Joystick Holding Tab (Autodesk Fusion 360 design; units mm, degrees)
Autodesk Fusion 360 part; units mm, degrees
sketch "Sketch1" plane through (0, 0, 0) normal (0, 0, 1) x (1, 0, 0)
  line L0 (0, 0) -> (30, 0)
  line L1 (30, 0) -> (30, -10)
  line L2 (30, -10) -> (0, -10)
  line L3 (0, -10) -> (0, 0)
  line L4 (25, 0) -> (25, -10)
  line L5 (0, 10) -> (0, 20)
  line L6 (15, 10) -> (0, 10)
  line L7 (0, 20) -> (15, 20)
  line L8 (15, 20) -> (15, 10)
  line L9 (10, 20) -> (10, 10)
  dimension "d1" = 30
  dimension "d2" = 10
  dimension "d3" = 5
  dimension "d12" = 15
  dimension "d13" = 10
  dimension "d14" = 5
  constraint horizontal L0
  constraint vertical L1
  constraint horizontal L2
  constraint vertical L3
  constraint coincident L0.start L3.end
  constraint coincident L0 L4.start
  constraint coincident L2 L4.end
  constraint perpendicular L2 L4
  constraint horizontal L7
  constraint vertical L8
  constraint horizontal L6
  constraint vertical L5
  constraint coincident L9.start L7
  constraint coincident L9.end L6
  constraint perpendicular L6 L9
  measures "d1" distance of L0.start L0.end
  measures "d2" distance of L0.start L2.end
  measures "d3" distance of L1 L4
  measures "d12" distance of L7.end L5.end
  measures "d13" distance of L5.end L5.start
  measures "d14" distance of L8 L9
extrude "Extrude1" add sketch "Sketch1" along normal blind 3.6 contours L0 L2 L3 L4 makes body 1
extrude "Extrude2" add sketch "Sketch1" along normal blind 10 contours L0 L1 L2 L4 bodies 1
fillet "Fillet1" radius 2 2 edges at (0, -10, 1.8) (0, 0, 1.8) on bodies 1
fillet "Fillet2" radius 2 2 edges at (27.5, 0, 10) (27.5, -10, 10) on bodies 1
extrude "Extrude3" add sketch "Sketch1" along normal blind 10 separate body contours L6 L7 L8 L9 makes body 2
extrude "Extrude4" add sketch "Sketch1" along normal blind 3.6 contours L5 L6 L7 L9 bodies 2
fillet "Fillet3" radius 2 4 edges at (12.5, 10, 10) (12.5, 20, 10) (0, 10, 1.8) (0, 20, 1.8) on bodies 2
